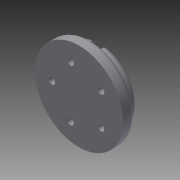
# Autodesk Inventor part: motorSupportNew1
Saved by Autodesk Inventor 2014 SP2 (Build 180246200, 246)
## iProperties
Created: 2020-04-08
Part Number: motorSupportNew1
Material: Generic
Document SubType Name: Sheet Metal
Designer: GauchoHP
Density: 1 g/cm^3
Sheet Metal Rule: Default_mm
Appearance: Default
Author: GauchoHP
Autodesk Inventor part; units mm, degrees
ref_plane "YZ Plane" through (0, 0, 0) normal (1, 0, 0) x (0, 1, 0)
ref_plane "XZ Plane" through (0, 0, 0) normal (0, 1, 0) x (-1, 0, 0)
ref_plane "XY Plane" through (0, 0, 0) normal (0, 0, 1) x (1, 0, 0)
sketch "Sketch1" plane through (0, 0, 0) normal (0, 1, 0) x (-1, 0, 0)
  circle A0 centre (0, 0) radius 18
  line L0 (10.3065, -1.0922) -> (4.2236, -9.4646)
  line L1 (2.1462, -10.1396) -> (-7.6962, -6.9416)
  line L2 (-8.9801, -5.1744) -> (-8.9801, 5.1744)
  line L3 (-7.6962, 6.9416) -> (2.1462, 10.1396)
  line L4 (4.2236, 9.4646) -> (10.3065, 1.0922)
  circle A1 centre (3.4301, 10.5567) radius 1.35
  circle A2 centre (11.1, 0) radius 1.35
  circle A3 centre (-8.9801, 6.5244) radius 1.35
  circle A4 centre (-8.9801, -6.5244) radius 1.35
  circle A5 centre (3.4301, -10.5567) radius 1.35
  arc A6 (11.0179, 1.3475) -> (4.6863, 10.0622) centre (0, 0) ccw
  arc A7 (4.6863, -10.0622) -> (11.0179, -1.3475) centre (0, 0) ccw
  arc A8 (-8.1216, -7.5663) -> (2.1232, -10.8951) centre (0, 0) ccw
  arc A9 (2.1232, 10.8951) -> (-8.1216, 7.5663) centre (0, 0) ccw
  arc A10 (-9.7057, 5.386) -> (-9.7057, -5.386) centre (0, 0) ccw
  dimension "d0" = 36
  dimension "d2" = 2.7
  dimension "d3" = 2.7
  dimension "d4" = 2.7
  dimension "d5" = 2.7
  dimension "d6" = 2.7
  constraints: 30 point on circle, 11 centre point, 10 end point, 3 coincident, 6 other
  measures "d0" diameter of A0
  measures "d2" diameter of A1
  measures "d3" diameter of A2
  measures "d4" diameter of A3
  measures "d5" diameter of A4
  measures "d6" diameter of A5
extrude "Extrusion1" add sketch "Sketch1" along normal blind 5 contours A0 | A2 A7 A5 L0 | L0 A5 L1 A4 L2 A3 L3 A1 L4 A2 | L4 A1 A6 A2 | A5 A8 A4 L1 | L3 A3 A9 A1 | A10 A3 L2 A4
sketch "Sketch2" plane through (0, 5, 0) normal (0, 1, 0) x (1, 0, 0)
  circle A0 centre (-11.1, 0) radius 1.35 projected
  circle A1 centre (8.9801, -6.5244) radius 1.35 projected
  circle A2 centre (8.9801, 6.5244) radius 1.35 projected
  circle A3 centre (0, 0) radius 18 projected
  circle A4 centre (0, 0) radius 15
  line L0 (2.5, 14.7902) -> (2.5, -14.7902)
  line L1 (-2.5, -14.7902) -> (-2.5, 14.7902)
  line L2 (-2.5, 2.5) -> (2.5, 2.5)
  line L3 (2.5, 2.5) -> (2.5, -2.5)
  line L4 (2.5, -2.5) -> (-2.5, -2.5)
  line L5 (-2.5, -2.5) -> (-2.5, 2.5)
  dimension "d9" = 30
  dimension "d11" = 2.5
  dimension "d16" = 2.5
  dimension "d17" = 5
  dimension "d18" = 5
  dimension "d19" = 0
  dimension "d20" = 2.5
  constraints: 12 end point, 4 point on circle, 3 parallel, 1 centre point, 1 coincident, 1 horizontal, 1 perpendicular
  measures "d9" diameter of A4
  measures "d11" distance from line of L1 A4.centre
  measures "d16" distance from line of A3.centre L0
  measures "d17" distance of L3.end L4.end
  measures "d18" distance of L2.end L3.end
  measures "d19" distance between parallel lines of L1 L5
  measures "d20" distance from line of A3.centre L2
extrude "Extrusion2" add sketch "Sketch2" along normal blind 4 contours A0 | A1 | A2 | A4 L0 | L1 A4 | L0 L4 L1 L2
fillet "Fillet1" radius 2 1 edges at (18, 5, 0)
fillet "Fillet2" radius 2 2 edges at (-15, 9, 0) (15, 9, 0)
equation "\"BendRadius\" = Thickness"
equation "\"BendReliefWidth\" = Thickness"
equation "\"BendReliefDepth\" = 0.5 * Thickness"
equation "\"CornerReliefSize\" = 4 * Thickness"
equation "\"MinimumRemnant\" = 2 * Thickness"
equation "\"TransitionRadius\" = BendRadius"
equation "\"JacobiRadiusSize\" = BendRadius"
equation "\"GapSize\" = Thickness"
equation "\"Thickness\" = 0.5"
body "Solid1"
